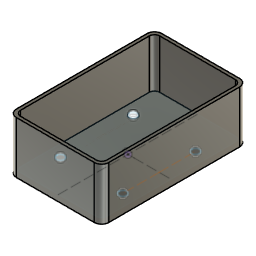
WeightBox Robotics (Autodesk Fusion 360 design; units mm, degrees)
Autodesk Fusion 360 part; units mm, degrees
note: some values were not read from the file. Set by a fixed rule: which face or edge a step refers to.
sketch "Sketch1" plane through (0, 0, 0) normal (0, 0, 1) x (1, 0, 0)
  line L0 (22.25, 35) -> (-22.25, 35)
  line L1 (-22.25, 35) -> (-22.25, -35)
  line L2 (-22.25, -35) -> (22.25, -35)
  line L3 (22.25, -35) -> (22.25, 35)
  line L4 (22.25, 35) -> (-22.25, -35) construction
  line L5 (-22.25, 35) -> (22.25, -35) construction
  dimension "d1" = 44.5
  dimension "d2" = 70
  constraint horizontal L0
  constraint perpendicular L0 L1
  constraint parallel L0 L2
  constraint parallel L1 L3
  constraint coincident L4 origin
  constraint coincident L5 origin
  measures "d1" distance of L1.end L2.end
  measures "d2" distance of L0.end L1.end
extrude "Extrude1" add sketch "Sketch1" along normal blind 25
shell "Shell1" thickness 1.5 removed faces 1 at (-7.4167, 11.6667, 25)
fillet "Fillet1" radius 3.5 4 edges at (22.25, 35, 12.5) (-22.25, 35, 12.5) (22.25, -35, 12.5) (-22.25, -35, 12.5)
fillet "Fillet2" radius 2.5 4 edges at (20.75, -33.5, 13.25) (-20.75, -33.5, 13.25) (-20.75, 33.5, 13.25) (20.75, 33.5, 13.25)
sketch "Sketch2" plane through (0, 0, 1.5) normal (0, 0, 1) x (-1, 0, 0)
  arc A0 (-20.75, -31) -> (-18.25, -33.5) centre (-18.25, -31) ccw
  line L0 (-18.25, -33.5) -> (18.25, -33.5)
  arc A1 (18.25, -33.5) -> (20.75, -31) centre (18.25, -31) ccw
  line L1 (20.75, -31) -> (20.75, 31)
  arc A2 (20.75, 31) -> (18.25, 33.5) centre (18.25, 31) ccw
  line L2 (18.25, 33.5) -> (-18.25, 33.5)
  arc A3 (-18.25, 33.5) -> (-20.75, 31) centre (-18.25, 31) ccw
  line L3 (-20.75, 31) -> (-20.75, -31)
  line L4 (0, 0) -> (-2.9788, 0) construction
  line L5 (-2.9788, 0) -> (-20.75, 0) construction
  line L6 (0, 33.5) -> (0, -33.5) construction
  line L7 (-15, 0) -> (-15, -17.5) construction
  line L8 (-15, 0) -> (-15, 17.5) construction
  circle A4 centre (-15, 17.5) radius 1.75
  circle A5 centre (-15, -17.5) radius 1.75
  circle A6 centre (15, 17.5) radius 1.75
  circle A7 centre (15, -17.5) radius 1.75
  dimension "d12" = 17.5
  dimension "d13" = 17.5
  dimension "d14" = 3.5
  dimension "d15" = 3.5
  constraint coincident L4.start origin
  constraint perpendicular L3 L4
  constraint midpoint L3 L5.end
  constraint perpendicular L3 L5
  constraint midpoint L2 L6.start
  constraint midpoint L0 L6.end
  constraint coincident L5 L7.start
  constraint perpendicular L5 L7
  constraint perpendicular L5 L8
  constraint coincident L8.end A4.centre
  constraint coincident L7.end A5.centre
  constraint symmetric L6 A4 A6
  constraint symmetric L6 A5 A7
  measures "d12" distance of L7.start L7.end
  measures "d13" distance of L7.start L8.end
  measures "d14" diameter of A4
  measures "d15" diameter of A5
extrude "Extrude2" cut sketch "Sketch2" against normal blind 40 contours A4 | A5
extrude "Extrude3" cut sketch "Sketch2" against normal blind 40 contours A4 | A5 | A6 | A7
chamfer "Chamfer1" distance 0.5 angle 45 4 edges at (-13.3684, 16.8672, 1.5) (-13.3684, -18.1328, 1.5) (16.6316, 16.8672, 1.5) (16.6316, -18.1328, 1.5)
thread "Thread1" "ISO Metric profile 3.5 M3.5x0.6 M3.5x0.6 6H" major diameter 3.5995 minor diameter 2.93 pitch 0.6 angle 60 resizes the face on face at (-16.7413, 17.6742, 0.6667)
thread "Thread2" "ISO Metric profile 3.5 M3.5x0.6 M3.5x0.6 6H" major diameter 3.5995 minor diameter 2.93 pitch 0.6 angle 60 resizes the face on face at (-16.7478, -17.4128, 0.3333)
thread "Thread3" "ISO Metric profile 3.5 M3.5x0.6 M3.5x0.6 6H" major diameter 3.5995 minor diameter 2.93 pitch 0.6 angle 60 resizes the face on face at (13.2522, 17.5872, 0.3333)
thread "Thread4" "ISO Metric profile 3.5 M3.5x0.6 M3.5x0.6 6H" major diameter 3.5995 minor diameter 2.93 pitch 0.6 angle 60 resizes the face on face at (13.2522, -17.4128, 0.3333)
